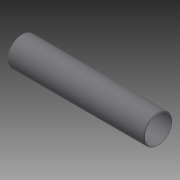
# Autodesk Inventor part: 17R-7.30250C
Saved by Autodesk Inventor 2014 (Build 180170000, 170)
## iProperties
Created: 2014-01-18
Part Number: 17R-7.30250C
Material: Generic
Catalog Web Link: www.cadenas.de
Description: Tube-Original Line - Standard Air Cylinders
Vendor: BIMBA
Document SubType Name: Standard Catalog Part
Designer: Andrew Toennies
Manufacturer: BIMBA
Density: 1 g/cm^3
Appearance: RGB(180.00000447034725,180.00000447034725,180.00000447034725)
Category: PARTsolutions
Company: BIMBA
Title: 17R-7.30250C
Author: Cadenas PARTsolutions
Comments: Original Line - Standard Air Cylinders
PSOL_IDENT_0: {$CADENAS_DATA\23d-libs\bimba\bimba\bimba_imperial\bimba_full_line\original_line_cylinders\standard_
PSOL_IDENT_1: air_cylinders\tube.prj},192 {VTYP=3D},{NB=17R-7.30250C},{LINA=17R-7.30250C},{NN=Tube},{DATE=20.08.20
PSOL_IDENT_2: 11 07:16:50},{GEOMDATE=18.02.2011 00:00:00},{VERSION=},{LINEID=80},{LINESUBID=-1},{WBVAR=MNT,ACTING,
PSOL_IDENT_3: NR,L,FOURHOLES,SR}  {NB=17R-7.30250C},{LINA=17R-7.30250C},{KT=DUMMY},{PN=17R-7.30250C},{BORE=1.50000
PSOL_IDENT_4: 000},{BOREPN=17},{MNT=},{MNTALG='' , 'Front Nose' , 'BF' , 'Front Block' , 'BFT' , 'Front Trunnion'
PSOL_IDENT_5: , 'A' , 'Adjustable Stroke'},{ACTING=R},{ACTINGALG= '' , 'Single Acting' , 'R' , 'Reverse/Double Act
PSOL_IDENT_6: ing' },{NR=},{NRALG= '' , 'Without Non-rotating Rod' , 'NR' , 'With Non-rotating Rod' },{L=7.3025},{
PSOL_IDENT_7: OD=1.5565},{ODN=1.5565},{ODP=1.5565},{ODB=1.5800},{ID=1.5115},{DV=0.00000000},{LV=0.00000000},{LV1=0
PSOL_IDENT_8: .00000000},{G=0.0400},{FOURHOLES=0},{AA=0.3750},{BB=0.1250},{SR=C},{SRALG= 'C' , 'Carbon Steel Rod'
PSOL_IDENT_9: , 'SR' , '303 Stainless Steel Rod' , '' , '303 Stainless Steel Rod'}
CNS_NN: Tube
CNS_NT: Original Line - Standard Air Cylinders
CNS_NB: 17R-7.30250C
CNS_NBSYN: $PN.
CNS_LINA: 17R-7.30250C
CNS_PN: 17R-7.30250C
CNS_BORE: 1 1/2
CNS_BOREPN: 17
CNS_MNT: Front Nose
CNS_MNTALG: '' , 'Front Nose' , 'BF' , 'Front Block' , 'BFT' , 'Front Trunnion' , 'A' , 'Adjustable Stroke'
CNS_ACTING: Reverse/Double Acting
CNS_ACTINGALG: '' , 'Single Acting' , 'R' , 'Reverse/Double Acting'
CNS_NR: Without Non-rotating Rod
CNS_NRALG: '' , 'Without Non-rotating Rod' , 'NR' , 'With Non-rotating Rod'
CNS_L: 7.3025
CNS_OD: 1.5565
CNS_ODN: 1.5565
CNS_ODP: 1.5565
CNS_ODB: 1.5800
CNS_ID: 1.5115
CNS_DV: 0.00000000
CNS_LV: 0.00000000
CNS_LV1: 0.00000000
CNS_G: 0.0400
CNS_FOURHOLES: 0
CNS_AA: 0.3750
CNS_BB: 0.1250
CNS_SR: Carbon Steel Rod
CNS_SRALG: 'C' , 'Carbon Steel Rod' , 'SR' , '303 Stainless Steel Rod' , '' , '303 Stainless Steel Rod'
SUPPLIER: BIMBA
ARTICLENO: 17R-7.30250C
BOMINFO: 17R-7.30250C
CREATOR: CADENAS GmbH
Autodesk Inventor part; units mm, degrees
ref_plane "YZ Plane" through (0, 0, 0) normal (1, 0, 0) x (0, 1, 0)
ref_plane "XZ Plane" through (0, 0, 0) normal (0, 1, 0) x (-1, 0, 0)
ref_plane "XY Plane" through (0, 0, 0) normal (0, 0, 1) x (1, 0, 0)
sketch "Sketch_1" plane through (0, 0, 0) normal (0, 0, 1) x (1, 0, 0)
  line L0 (185.4835, 0) -> (0, 0)
  arc A0 (-0.8826, 18.7343) -> (-0.8826, 18.5547) centre (-0.7928, 18.6445) ccw
  line L1 (-0.8826, 18.5547) -> (-0.508, 18.1801)
  line L2 (-0.508, 18.1801) -> (0, 18.1801)
  line L3 (0, 18.1801) -> (1.016, 19.196)
  line L4 (1.016, 19.196) -> (184.4675, 19.196)
  line L5 (184.4675, 19.196) -> (185.4835, 18.1801)
  line L6 (185.4835, 18.1801) -> (185.9915, 18.1801)
  line L7 (185.9915, 18.1801) -> (186.3661, 18.5547)
  arc A1 (186.3661, 18.5547) -> (186.3661, 18.7343) centre (186.2763, 18.6445) ccw
  line L8 (186.3661, 18.7343) -> (185.6304, 19.47)
  arc A2 (185.6304, 19.47) -> (184.912, 19.7675) centre (184.912, 18.7515) ccw
  line L9 (184.912, 19.7675) -> (0.5715, 19.7675)
  arc A3 (0.5715, 19.7675) -> (-0.1469, 19.47) centre (0.5715, 18.7515) ccw
  line L10 (-0.1469, 19.47) -> (-0.8826, 18.7343)
  constraints: 22 end point, 8 point on circle, 4 centre point
revolve "Revolution1" add sketch "Sketch_1" angle 360 about axis through (185.4835, 0, 0) along (1, 0, 0)
ref_plane "cp1_XY" through (92.7417, 19.7675, 0) normal (1, 0, 0) x (0, 0, -1)
ref_plane "cp1_YZ" through (92.7417, 19.7675, 0) normal (0, 0, -1) x (0, 1, 0)
ref_plane "cp1_ZX" through (92.7417, 19.7675, 0) normal (0, 1, 0) x (1, 0, 0)
ref_plane "cp2_XY" through (92.7417, 0, -19.7675) normal (1, 0, 0) x (0, 0, -1)
ref_plane "cp2_YZ" through (92.7417, 0, -19.7675) normal (0, 0, -1) x (0, 1, 0)
ref_plane "cp2_ZX" through (92.7417, 0, -19.7675) normal (0, 1, 0) x (1, 0, 0)
ref_plane "cp3_XY" through (92.7417, -19.7675, 0) normal (1, 0, 0) x (0, 0, -1)
ref_plane "cp3_YZ" through (92.7417, -19.7675, 0) normal (0, 0, -1) x (0, 1, 0)
ref_plane "cp3_ZX" through (92.7417, -19.7675, 0) normal (0, 1, 0) x (1, 0, 0)
ref_plane "cp4_XY" through (92.7417, 0, 19.7675) normal (1, 0, 0) x (0, 0, -1)
ref_plane "cp4_YZ" through (92.7417, 0, 19.7675) normal (0, 0, -1) x (0, 1, 0)
ref_plane "cp4_ZX" through (92.7417, 0, 19.7675) normal (0, 1, 0) x (1, 0, 0)
ref_plane "tube_front_XY" through (0, 0, 0) normal (1, 0, 0) x (0, 0, -1)
ref_plane "tube_front_YZ" through (0, 0, 0) normal (0, 0, -1) x (0, 1, 0)
ref_plane "tube_front_ZX" through (0, 0, 0) normal (0, 1, 0) x (1, 0, 0)
ref_plane "tube_rear_XY" through (185.4835, 0, 0) normal (1, 0, 0) x (0, 0, -1)
ref_plane "tube_rear_YZ" through (185.4835, 0, 0) normal (0, 0, -1) x (0, 1, 0)
ref_plane "tube_rear_ZX" through (185.4835, 0, 0) normal (0, 1, 0) x (1, 0, 0)
body "Solid1"
